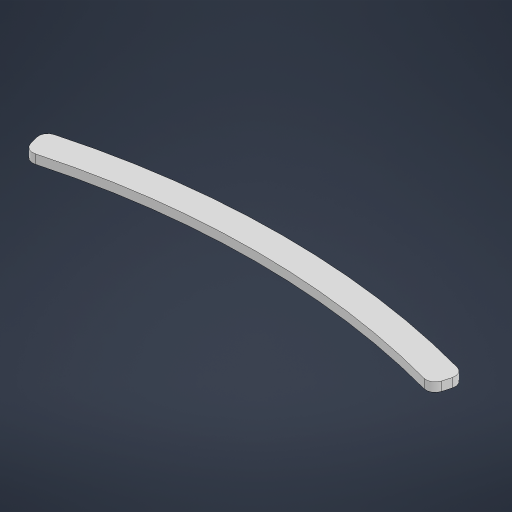
# Autodesk Inventor part: SubHandle
Saved by Autodesk Inventor 2024.2 (Build 282272000, 272)
## iProperties
Created: 2023-12-29
Part Number: SubHandle
Material: 一般
Document SubType Name: Modeling
Designer: Hanaoka
Density: 1 g/cm^3
Appearance: 既定
Author: Hanaoka
Autodesk Inventor part; units mm, degrees
ref_plane "YZ Plane" through (0, 0, 0) normal (1, 0, 0) x (0, 1, 0)
ref_plane "XZ Plane" through (0, 0, 0) normal (0, 1, 0) x (-1, 0, 0)
ref_plane "XY Plane" through (0, 0, 0) normal (0, 0, 1) x (1, 0, 0)
sketch "スケッチ1" plane through (0, 0, 0) normal (0, 1, 0) x (-1, 0, 0)
  arc A0 (-44.6969, -164.0189) -> (44.6969, -164.0189) centre (0, 0) ccw
  arc A1 (-43.0967, -158.2361) -> (43.0967, -158.2361) centre (0, 0) ccw
  line L0 (45.5455, -159.6171) -> (46.0943, -161.5404)
  line L1 (-45.5455, -159.6171) -> (-46.0943, -161.5404)
  arc A2 (44.6969, -164.0189) -> (46.0943, -161.5404) centre (44.1711, -162.0892) ccw
  arc A3 (45.5455, -159.6171) -> (43.0967, -158.2361) centre (43.6222, -160.1659) ccw
  arc A4 (-43.0967, -158.2361) -> (-45.5455, -159.6171) centre (-43.6222, -160.1659) ccw
  arc A5 (-46.0943, -161.5404) -> (-44.6969, -164.0189) centre (-44.1711, -162.0892) ccw
  line L2 (0, -204) -> (0, 34) projected
  point P0 (-46.6463, -163.4751)
  point P1 (46.6463, -163.4751)
  point P2 (-45, -157.7054)
  point P3 (45, -157.7054)
  point P4 (-46.6463, -163.4751)
  dimension "d0" = 170
  dimension "d1" = 6
  dimension "d2" = 2
  dimension "d3" = 90
  constraints: 17 point on circle, 8 tangent, 6 centre point, 5 point on line, 4 end point, 4 line through centre, 3 equal radius, 2 coincident, 1 other
  measures "d0" radius of A0
  measures "d1" radial gap between concentric circles of A0 A1
  measures "d2" radius of A2
  measures "d3" distance of point (-45, -157.705) point (45, -157.705)
extrude "押し出し1" add sketch "スケッチ1" along normal blind 2
